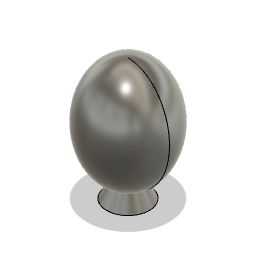
balloon (Autodesk Fusion 360 design; units mm, degrees)
Autodesk Fusion 360 part; units mm, degrees
sketch "Sketch1" plane through (0, 0, 0) normal (0, 0, 1) x (1, 0, 0)
  line L0 (0, 0) -> (12.5, 0)
  line L1 (12.5, 0) -> (12.5, 36)
  line L2 (12.5, 36) -> (0, 36)
  line L3 (0, 36) -> (0, 0)
  line L4 (3, 0) -> (3, 36) construction
  line L5 (4, 0) -> (4, 36) construction
  line L6 (0, 4.2) -> (12.5, 4.2) construction
  line L7 (4, 4.2) -> (6.4249, 0)
  line L8 (4, 4.2) -> (8.8497, 4.2) construction
  line L9 (0, 36) -> (0, 0)
  line L10 (0, 36) -> (0, 36.6648)
  ellipse E0 centre (0, 20) end of major axis (12.5, 20) minor radius 16.6648 (0, 3.3352) -> (0, 36.6648) ccw
  line L11 (4, 4.2) -> (4, 4.2115)
  dimension "d1" = 12.5
  dimension "d2" = 36
  dimension "d3" = 3
  dimension "d4" = 4
  dimension "d5" = 4.2
  dimension "d6" = 60
  constraint horizontal L0
  constraint vertical L1
  constraint horizontal L2
  constraint vertical L3
  constraint coincident L0.start L3.end
  constraint coincident L0 L4.start
  constraint coincident L2 L4.end
  constraint perpendicular L2 L4
  constraint coincident L0 L5.start
  constraint coincident L2 L5.end
  constraint perpendicular L2 L5
  constraint coincident L3 L6.start
  constraint coincident L1 L6.end
  constraint perpendicular L1 L6
  constraint horizontal L8
  constraint coincident L5 L7.start
  constraint coincident L6 L7.start
  constraint coincident L0 L7.end
  constraint coincident L9 E0.centre
  constraint coincident E0 L11.end
  constraint perpendicular L6 L11
  measures "d1" distance of L0.start L0.end
  measures "d2" distance of L0.start L2.end
  measures "d3" distance of L3 L4
  measures "d4" distance of L3 L5
  measures "d5" distance of L0 L6
  measures "d6" angle of L7 L8
sketch "Sketch2" plane through (0, 0, 0) normal (0, -1, 0) x (1, 0, 0)
  circle A0 centre (0, 0) radius 3.45
  circle A1 centre (0, 0) radius 6.4249
  dimension "d8" = 6.9
  constraint coincident A0.centre A1.centre
  measures "d8" diameter of A0
revolve "Revolve2" add sketch "Sketch1" angle 360 about axis through (0, 36, 0) along (0, -1, 0) contours L0 L3 L7 L9 E0 L11 | L2 L3 L9 E0 | L2 L10 E0
extrude "Extrude2" cut sketch "Sketch2" against normal blind 10 contours A0
